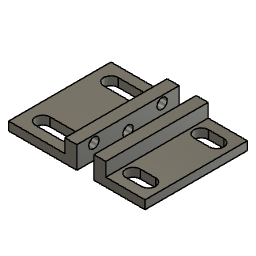
Curtain Clamps v2 (Autodesk Fusion 360 design; units mm, degrees)
Autodesk Fusion 360 part; units mm, degrees
sketch "Sketch1" plane through (0, 0, 0) normal (0, 1, 0) x (1, 0, 0)
  line L0 (20, 30) -> (-20, 30)
  line L1 (-20, 30) -> (-20, -30)
  line L2 (-20, -30) -> (20, -30)
  line L3 (20, -30) -> (20, 30)
  line L4 (20, 30) -> (-20, -30) construction
  line L5 (-20, 30) -> (20, -30) construction
  circle A0 centre (-10, 20) radius 4.25
  circle A1 centre (5, 20) radius 4.25
  circle A2 centre (-10, -20) radius 4.25
  circle A3 centre (5, -20) radius 4.25
  line L6 (-10, 15.75) -> (5, 15.75)
  line L7 (5, 15.75) -> (5, 24.25)
  line L8 (5, 24.25) -> (-10, 24.25)
  line L9 (-10, 24.25) -> (-10, 15.75)
  line L10 (-10, -24.25) -> (5, -24.25)
  line L11 (5, -24.25) -> (5, -15.75)
  line L12 (5, -15.75) -> (-10, -15.75)
  line L13 (-10, -15.75) -> (-10, -24.25)
  dimension "d1" = 40
  dimension "d2" = 60
  dimension "d3" = 8.5
  dimension "d4" = 8.5
  dimension "d5" = 8.5
  dimension "d6" = 8.5
  constraint horizontal L0
  constraint perpendicular L0 L1
  constraint parallel L0 L2
  constraint parallel L1 L3
  constraint coincident L4 origin
  constraint coincident L5 origin
  constraint perpendicular L6 L7
  constraint parallel L6 L8
  constraint parallel L7 L9
  constraint coincident A1 L6.end
  constraint tangent A1 L6
  constraint horizontal L6
  constraint coincident A0 L6.start
  constraint perpendicular L10 L11
  constraint parallel L10 L12
  constraint parallel L11 L13
  constraint coincident A3 L10.end
  constraint tangent A3 L10
  constraint perpendicular L9 L10
  constraint coincident A2 L10.start
  measures "d1" distance of L1.end L2.end
  measures "d2" distance of L0.end L1.end
  measures "d3" diameter of A0
  measures "d4" diameter of A1
  measures "d5" diameter of A2
  measures "d6" diameter of A3
extrude "Extrude1" add sketch "Sketch1" along normal blind 5 makes body 1
sketch "Sketch2" plane through (0, 5, 0) normal (0, 1, 0) x (-1, 0, 0)
  line L0 (10, 15.75) -> (-5, 15.75)
  arc A0 (-5, 24.25) -> (-5, 15.75) centre (-5, 20) ccw
  line L1 (-5, 24.25) -> (10, 24.25)
  arc A1 (10, 15.75) -> (10, 24.25) centre (10, 20) ccw
  line L2 (10, -24.25) -> (-5, -24.25)
  arc A2 (-5, -15.75) -> (-5, -24.25) centre (-5, -20) ccw
  line L3 (-5, -15.75) -> (10, -15.75)
  arc A3 (10, -24.25) -> (10, -15.75) centre (10, -20) ccw
  line L4 (-20, 30) -> (-20, -30)
  line L5 (-20, -30) -> (20, -30)
  line L6 (20, -30) -> (20, 30)
  line L7 (20, 30) -> (-20, 30)
  line L8 (-20, -30) -> (-13, -30)
  line L9 (-13, -30) -> (-13, 30)
  line L10 (-13, 30) -> (-20, 30)
  line L11 (-20, 30) -> (-20, -30)
  dimension "d9" = 7
  constraint horizontal L8
  constraint vertical L9
  constraint horizontal L10
  constraint vertical L11
  constraint coincident L4.end L5.start
  measures "d9" distance of L4.end L8.end
extrude "Extrude2" add sketch "Sketch2" along normal blind 8 contours L4 L5 L7 L8 L9 L10 L11 bodies 1
sketch "Sketch3" plane through (20, 0, 0) normal (1, 0, 0) x (0, 0, -1)
  line L0 (-30, 0) -> (30, 0)
  line L1 (30, 0) -> (30, 13)
  line L2 (30, 13) -> (-30, 13)
  line L3 (-30, 13) -> (-30, 0)
  circle A0 centre (-20, 9) radius 3
  circle A1 centre (0, 5) radius 3
  circle A2 centre (20, 9) radius 3
  dimension "d22" = 6
  dimension "d23" = 6
  dimension "d24" = 6
  measures "d22" diameter of A0
  measures "d23" diameter of A1
  measures "d24" diameter of A2
extrude "Extrude3" cut sketch "Sketch3" against normal blind 4 contours A0 | A1 | A2 bodies 1
sketch "Sketch4" plane through (0, 0, 0) normal (0, 1, 0) x (1, 0, 0)
  line L0 (30, 30) -> (60, 30)
  line L1 (60, 30) -> (60, -30)
  line L2 (60, -30) -> (30, -30)
  line L3 (30, -30) -> (30, 30)
  circle A0 centre (43, 20) radius 4.25
  circle A1 centre (43, -20) radius 4.25
  circle A2 centre (52, -20) radius 4.25
  circle A3 centre (52, 20) radius 4.25
  line L4 (43, 24.25) -> (52, 24.25)
  line L5 (52, 24.25) -> (52, 15.75)
  line L6 (52, 15.75) -> (43, 15.75)
  line L7 (43, 15.75) -> (43, 24.25)
  line L8 (43, -15.75) -> (52, -15.75)
  line L9 (52, -15.75) -> (52, -24.25)
  line L10 (52, -24.25) -> (43, -24.25)
  line L11 (43, -24.25) -> (43, -15.75)
  dimension "d18" = 8.5
  dimension "d19" = 8.5
  dimension "d29" = 8.5
  dimension "d30" = 8.5
  constraint horizontal L0
  constraint vertical L1
  constraint horizontal L2
  constraint vertical L3
  constraint horizontal L4
  constraint vertical L5
  constraint horizontal L6
  constraint vertical L7
  constraint coincident A3 L5.end
  constraint coincident A0 L4.start
  constraint horizontal L8
  constraint vertical L9
  constraint horizontal L10
  constraint vertical L11
  constraint coincident A2 L9.end
  constraint coincident A1 L8.start
  measures "d18" diameter of A0
  measures "d19" diameter of A1
  measures "d29" diameter of A2
  measures "d30" diameter of A3
extrude "Extrude4" add sketch "Sketch4" along normal blind 5 separate body makes body 2
sketch "Sketch5" plane through (0, 5, 0) normal (0, 1, 0) x (-1, 0, 0)
  line L0 (-30, 30) -> (-60, 30)
  line L1 (-60, 30) -> (-60, -30)
  line L2 (-60, -30) -> (-30, -30)
  line L3 (-30, -30) -> (-30, 30)
  line L4 (-30, -30) -> (-37, -30)
  line L5 (-37, -30) -> (-37, 30)
  line L6 (-37, 30) -> (-30, 30)
  line L7 (-30, 30) -> (-30, -30)
  arc A0 (-43, -24.25) -> (-43, -15.75) centre (-43, -20) ccw
  line L8 (-43, -24.25) -> (-52, -24.25)
  arc A1 (-52, -15.75) -> (-52, -24.25) centre (-52, -20) ccw
  line L9 (-52, -15.75) -> (-43, -15.75)
  arc A2 (-43, 15.75) -> (-43, 24.25) centre (-43, 20) ccw
  line L10 (-43, 15.75) -> (-52, 15.75)
  arc A3 (-52, 24.25) -> (-52, 15.75) centre (-52, 20) ccw
  line L11 (-52, 24.25) -> (-43, 24.25)
  constraint horizontal L4
  constraint vertical L5
  constraint horizontal L6
  constraint vertical L7
  constraint coincident L0 L5.end
  constraint coincident L2.end L3.start
extrude "Extrude5" add sketch "Sketch5" along normal blind 8 contours L0 L2 L3 L4 L5 L6 L7 bodies 2
extrude "Extrude6" cut sketch "Sketch3" along normal blind 14 contours A0 | A1 | A2 bodies 2
